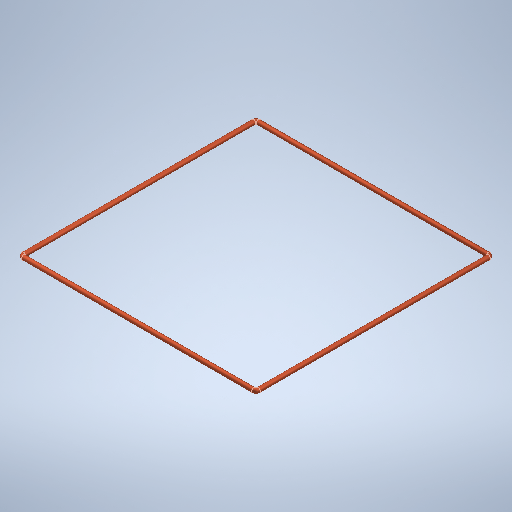
# Autodesk Inventor part: Coil_Of_Wire
Saved by Autodesk Inventor 2025 (Build 290162010, 162A)
## iProperties
Created: 2024-10-04
Part Number: Coil_Of_Wire
Material: Copper
Document SubType Name: Modeling
Designer: Tom
Density: 8.94 g/cm^3
Appearance: Copper - Satin
Author: Tom
Autodesk Inventor part; units mm, degrees
ref_plane "YZ Plane" through (0, 0, 0) normal (1, 0, 0) x (0, 1, 0)
ref_plane "XZ Plane" through (0, 0, 0) normal (0, 1, 0) x (-1, 0, 0)
sketch "Sketch1" plane through (0, 0, 0) normal (0, 1, 0) x (-1, 0, 0)
  line L0 (0, 0) -> (266.7, 0)
  line L1 (266.7, 0) -> (266.7, -266.7)
  line L2 (266.7, -266.7) -> (0, -266.7)
  line L3 (0, -266.7) -> (0, 0)
  line L4 (-2.5946, 0) -> (-2.5946, -266.7)
  line L5 (0, -269.2946) -> (266.7, -269.2946)
  line L6 (269.2946, -266.7) -> (269.2946, 0)
  line L7 (266.7, 2.5946) -> (0, 2.5946)
  arc A0 (-2.5946, -266.7) -> (0, -269.2946) centre (0, -266.7) ccw
  arc A1 (266.7, -269.2946) -> (269.2946, -266.7) centre (266.7, -266.7) ccw
  arc A2 (269.2946, 0) -> (266.7, 2.5946) centre (266.7, 0) ccw
  arc A3 (0, 2.5946) -> (-2.5946, 0) centre (0, 0) ccw
  dimension "d1" = 2.5946
  dimension "d2" = 2.5946
  dimension "d3" = 2.5946
  dimension "d4" = 2.5946
  dimension "d5" = 2.5946
  dimension "d7" = 266.7
  dimension "d8" = 2.5946
  constraints: 16 end point, 8 point on circle, 8 tangent, 5 perpendicular, 4 centre point, 2 equal radius, 2 parallel, 1 horizontal, 1 vertical
  measures "d1" distance between parallel lines of L3 L4
  measures "d2" distance between parallel lines of L2 L5
  measures "d3" distance between parallel lines of L1 L6
  measures "d4" distance between parallel lines of L7 L0
  measures "d5" radius of A0
  measures "d7" distance of L2.end L0.start
  measures "d8" radius of A3
ref_plane "Work Plane1" through (2.5946, 0, 0) normal (0, 0, -1) x (-1, 0, 0)
sketch "Sketch2" plane through (2.5946, 0, 0) normal (0, 0, -1) x (-1, 0, 0)
  circle A0 centre (0, 0) radius 2.5946
  point P0 (2.5946, 0)
  dimension "d9" = 5.1892
  constraints: 1 centre point
  measures "d9" diameter of A0
sweep "Sweep1" add profiles "Sketch2" path "Sketch1" path curves L4 A0 L5 A1 L6 A2 L7 A3
body "Solid1"
